Magnetabstander_v2 (Autodesk Fusion 360 design; units mm, degrees)
Autodesk Fusion 360 part; units mm, degrees
note: some values were not read from the file. Set by a fixed rule: which sketch regions a step uses.
sketch "Sketch1" plane through (0, 0, 0) normal (0, 1, 0) x (1, 0, 0)
  circle A0 centre (0, 0) radius 19.5
  circle A1 centre (0, 0) radius 13
  line L0 (-21.8994, 0) -> (35, 0)
  circle A2 centre (-13, 0) radius 5.3
  circle A3 centre (13, 0) radius 5.3
  circle A4 centre (6.5, 11.2583) radius 5.3
  circle A5 centre (6.5, -11.2583) radius 5.3
  dimension "d1" = 39
  dimension "d2" = 26
  dimension "d3" = 10.6
  dimension "d4" = 10.6
  dimension "d7" = 10.6
  dimension "d8" = 10.6
  constraint coincident A0.centre A1.centre
  constraint horizontal L0
  constraint coincident L0 A2.centre
  constraint coincident A1 A2.centre
  constraint coincident A1 A3.centre
  constraint coincident L0 A3.centre
  measures "d1" diameter of A0
  measures "d2" diameter of A1
  measures "d3" diameter of A2
  measures "d4" diameter of A3
  measures "d7" diameter of A4
  measures "d8" diameter of A5
extrude "Extrude1" add sketch "Sketch1" along normal blind 1.2 contours A0 A1 L0 A2 A3 A4 | A0 A1 L0 A2 A3 A5 | A1 L0 A2 A3 A4 | A1 L0 A2 A3 A5 | A1 A4 | A1 A4 | A1 A5 | A1 A5 makes body 1
extrude "Extrude2" add sketch "Sketch1" along normal blind 1.2 separate body contours A0 A1 L0 A2 A3 A4 | A0 A1 L0 A2 A3 A5 | A1 L0 A3 | A1 L0 A3 | A1 L0 A3 | A1 L0 A3 | A1 L0 A2 A3 A4 | A1 L0 A2 A3 A5 makes body 2
